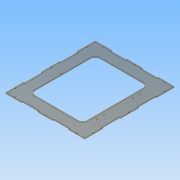
# Autodesk Inventor part: крышка
Saved by Autodesk Inventor 2017 (Build 210142000, 142)
## iProperties
Part Number: крышка
Material: Типовые
Document SubType Name: Modeling
Designer: Max
Mass: 263.553 g
Surface Area: 1424.23 cm^2
Volume: 263.553 cm^3
Density: 1 g/cm^3
Appearance: Поликарбонат — дымчатый
Author: Max
Autodesk Inventor part; units mm, degrees
ref_plane "YZ Plane" through (0, 0, 0) normal (1, 0, 0) x (0, 1, 0)
ref_plane "XZ Plane" through (0, 0, 0) normal (0, 1, 0) x (-1, 0, 0)
ref_plane "XY Plane" through (0, 0, 0) normal (0, 0, 1) x (1, 0, 0)
sketch "Эскиз1" plane through (0, 0, 0) normal (0, 0, 1) x (1, 0, 0)
  line L0 (46, -47) -> (277, -47)
  line L1 (277, -47) -> (277, -333)
  line L2 (277, -333) -> (46, -333)
  line L3 (46, -333) -> (46, -47)
  line L4 (-2, 5) -> (334, 5) projected
  line L5 (338, 5) -> (338, -385) projected
  line L6 (334, -385) -> (-2, -385) projected
  line L7 (-6, -385) -> (-6, 5) projected
  line L8 (-6, 5) -> (338, 5)
  line L9 (338, 5) -> (338, -385)
  line L10 (338, -385) -> (-6, -385)
  line L11 (-6, -385) -> (-6, 5)
  dimension "d4" = 231
  dimension "d10" = 61
  dimension "d11" = 52
  dimension "d12" = 52
  dimension "d13" = 52
  constraints: 16 end point, 4 parallel, 2 horizontal, 2 perpendicular
  measures "d4" distance between parallel lines of L1 L3
  measures "d10" distance between parallel lines of L5 L1
  measures "d11" distance between parallel lines of L4 L0
  measures "d12" distance between parallel lines of L6 L2
  measures "d13" distance between parallel lines of L7 L3
extrude "Выдавливание3" add sketch "Эскиз1" along normal blind 4
sketch "Эскиз3" plane through (0, 0, 4) normal (0, 0, 1) x (1, 0, 0)
  circle A0 centre (290.75, -97) radius 1.5
  circle A1 centre (290.75, -127) radius 1.5
  line L0 (46, -47) -> (277, -47) projected
  line L1 (277, -47) -> (277, -333) projected
  circle A2 centre (290.75, -253) radius 1.5
  circle A3 centre (290.75, -283) radius 1.5
  line L2 (277, -333) -> (46, -333) projected
  point P0 (0, 0)
  dimension "d19" = 3
  dimension "d20" = 3
  dimension "d21" = 30
  dimension "d22" = 50
  dimension "d23" = 13.75
  dimension "d24" = 13.75
  dimension "d25" = 3
  dimension "d26" = 3
  dimension "d27" = 30
  dimension "d28" = 13.75
  dimension "d29" = 13.75
  dimension "d30" = 50
  constraints: 4 centre point
  measures "d19" diameter of A0
  measures "d20" diameter of A1
  measures "d21" distance of A1.centre A0.centre
  measures "d22" distance from line of L0 A0.centre
  measures "d23" distance from line of L1 A0.centre
  measures "d24" distance from line of L1 A1.centre
  measures "d25" diameter of A2
  measures "d26" diameter of A3
  measures "d27" distance of A3.centre A2.centre
  measures "d28" distance from line of L1 A2.centre
  measures "d29" distance from line of L1 A3.centre
  measures "d30" distance from line of L2 A3.centre
extrude "Выдавливание4" cut sketch "Эскиз3" against normal blind 10
chamfer "Фаска1" distance 15 angle 45 4 edges at (277, -47, 2) (277, -333, 2) (46, -47, 2) (46, -333, 2)
sketch "Эскиз4" plane through (0, 0, 4) normal (0, 0, 1) x (1, 0, 0)
  ellipse E0 centre (40.9735, -191.8546) end of major axis (40.9735, -190.3546) minor radius 1.4997 projected
  line L0 (40.9735, -191.8546) -> (10.6659, -191.8546) construction
  circle A0 centre (40.733, -191.8546) radius 1.5
  line L1 (46, -62) -> (46, -318) projected
  point P0 (0, 0)
  dimension "d36" = 3
  dimension "d37" = 5.267
  constraints: 2 end point, 1 centre point, 1 horizontal, 1 point on line, 1 other
  measures "d36" diameter of A0
  measures "d37" distance from line of L1 A0.centre
extrude "Выдавливание5" cut sketch "Эскиз4" against normal blind 10 contours A0 E0 | E0 A0 picked at (41.2979, -191.9775) picked at (39.4227, -191.6148)
sketch "Эскиз5" plane through (0, 0, 4) normal (0, 0, 1) x (1, 0, 0)
  line L0 (-6, -73.3) -> (-2, -73.3) projected
  line L1 (-6, -150.7) -> (-2, -150.7) projected
  line L2 (-2, -73.3) -> (-2, -150.7) projected
  line L3 (-6, 5) -> (-6, -385) projected
  line L4 (-6, -229.3) -> (-2, -229.3) projected
  line L5 (-2, -229.3) -> (-2, -306.7) projected
  line L6 (-6, -306.7) -> (-2, -306.7) projected
  line L7 (63.3, -385) -> (63.3, -381) projected
  line L8 (133.2, -385) -> (63.3, -385) projected
  line L9 (133.2, -385) -> (133.2, -381) projected
  line L10 (63.3, -381) -> (133.2, -381) projected
  line L11 (63.3, -385) -> (63.3, -381) projected
  line L12 (268.7, -385) -> (198.8, -385) projected
  line L13 (268.7, -385) -> (268.7, -381) projected
  line L14 (198.8, -381) -> (268.7, -381) projected
  line L15 (198.8, -385) -> (198.8, -381) projected
  line L16 (63.3, 5) -> (133.2, 5) projected
  line L17 (63.3, 5) -> (63.3, 1) projected
  line L18 (133.2, 1) -> (63.3, 1) projected
  line L19 (133.2, 5) -> (133.2, 1) projected
  line L20 (198.8, 5) -> (268.7, 5) projected
  line L21 (198.8, 5) -> (198.8, 1) projected
  line L22 (268.7, 1) -> (198.8, 1) projected
  line L23 (268.7, 5) -> (268.7, 1) projected
  line L24 (338, -229.3) -> (334, -229.3) projected
  line L25 (334, -306.7) -> (334, -229.3) projected
  line L26 (338, -306.7) -> (334, -306.7) projected
  line L27 (338, -229.3) -> (338, -306.7) projected
  line L28 (338, -150.7) -> (334, -150.7) projected
  line L29 (338, -73.3) -> (338, -150.7) projected
  line L30 (334, -150.7) -> (334, -73.3) projected
  line L31 (338, -73.3) -> (334, -73.3) projected
  line L32 (63.1, 0.8) -> (63.1, 5.2)
  line L33 (63.1, 5.2) -> (133.4, 5.2)
  line L34 (133.4, 5.2) -> (133.4, 0.8)
  line L35 (133.4, 0.8) -> (63.1, 0.8)
  line L36 (198.6, 0.8) -> (198.6, 5.2)
  line L37 (198.6, 5.2) -> (268.9, 5.2)
  line L38 (268.9, 5.2) -> (268.9, 0.8)
  line L39 (268.9, 0.8) -> (198.6, 0.8)
  line L40 (333.8, -73.1) -> (333.8, -150.9)
  line L41 (333.8, -150.9) -> (338.2, -150.9)
  line L42 (338.2, -150.9) -> (338.2, -73.1)
  line L43 (338.2, -73.1) -> (333.8, -73.1)
  line L44 (333.8, -229.1) -> (338.2, -229.1)
  line L45 (338.2, -229.1) -> (338.2, -306.9)
  line L46 (338.2, -306.9) -> (333.8, -306.9)
  line L47 (333.8, -306.9) -> (333.8, -229.1)
  line L48 (268.9, -380.8) -> (268.9, -385.2)
  line L49 (268.9, -385.2) -> (198.6, -385.2)
  line L50 (198.6, -385.2) -> (198.6, -380.8)
  line L51 (198.6, -380.8) -> (268.9, -380.8)
  line L52 (133.2, -385) -> (63.3, -385) projected
  line L53 (133.2, -385) -> (133.2, -381) projected
  line L54 (63.3, -381) -> (133.2, -381) projected
  line L55 (63.3, -385) -> (63.3, -381) projected
  line L56 (63.3, -385) -> (63.3, -381) projected
  line L57 (63.3, -381) -> (133.2, -381) projected
  line L58 (-6, -306.9) -> (-1.8, -306.9)
  line L59 (-1.8, -306.9) -> (-1.8, -229.1)
  line L60 (-1.8, -229.1) -> (-6, -229.1)
  line L61 (-6, -150.9) -> (-1.8, -150.9)
  line L62 (-1.8, -150.9) -> (-1.8, -73.1)
  line L63 (-1.8, -73.1) -> (-6, -73.1)
  line L64 (-6, -73.1) -> (-6, -150.9)
  line L65 (-6, -229.1) -> (-6, -306.9)
  line L66 (63.3, -381) -> (133.2, -381)
  line L67 (133.2, -381) -> (133.2, -385)
  line L68 (133.2, -385) -> (63.3, -385)
  line L69 (63.3, -385) -> (63.3, -381)
  line L70 (63.3, -380.8) -> (133.2, -380.8)
  line L71 (63.1, -385) -> (63.1, -381)
  line L72 (133.4, -385) -> (133.4, -381)
  line L73 (133.4, -380.8) -> (63.1, -380.8)
  line L74 (63.1, -380.8) -> (63.1, -385.2)
  line L75 (63.1, -385.2) -> (133.4, -385.2)
  line L76 (133.4, -385.2) -> (133.4, -380.8)
  point P0 (0, 0)
  dimension "d40" = 4
  dimension "d41" = 69.9
  dimension "d42" = 69.9
  dimension "d43" = 0.2
  dimension "d44" = 0.2
  dimension "d45" = 0.2
  dimension "d46" = 0.2
  dimension "d47" = 0.2
  dimension "d48" = 0.2
  dimension "d49" = 0.2
  dimension "d50" = 0.2
  dimension "d51" = 0.2
  dimension "d52" = 0.2
  constraints: 78 end point, 7 parallel, 2 collinear, 2 horizontal, 2 perpendicular, 19 other
  measures "d40" distance between parallel lines of L18 L16
  measures "d41" distance between parallel lines of L19 L17
  measures "d42" distance between parallel lines of L23 L21
  measures "d43" distance between parallel lines of L18 L35
  measures "d44" distance between parallel lines of L21 L36
  measures "d45" distance between parallel lines of L30 L40
  measures "d46" distance between parallel lines of L25 L47
  measures "d47" distance between parallel lines of L14 L51
  measures "d48" distance between parallel lines of L6 L58
  measures "d49" distance between parallel lines of L1 L61
  measures "d50" distance between parallel lines of L10 L70
  measures "d51" distance between parallel lines of L7 L71
  measures "d52" distance between parallel lines of L9 L72
extrude "Выдавливание6" cut sketch "Эскиз5" against normal blind 4.2 contours L3 L63 L62 L61 L1 L2 L0 | L60 L59 L58 L3 L6 L5 L4 | L0 L2 L1 L3 | L4 L5 L6 L3 | L7 L10 L9 L8 | L12 L15 L14 L13 | L16 L19 L18 L17 | L20 L23 L22 L21 | L27 L26 L25 L24 | L28 L30 L31 L29 | L32 L33 L34 L35 | L36 L37 L38 L39 | L43 L42 L41 L40 | L44 L45 L46 L47 | L48 L49 L50 L51 | L70 L73 L76 L72 L75 L74 L71
sketch "Эскиз6" plane through (0, 0, 4) normal (0, 0, 1) x (1, 0, 0)
  line L0 (302.85, -381) -> (302.85, -385) projected
  line L1 (299.85, -385) -> (299.85, -381) projected
  line L2 (167.5, -381) -> (167.5, -385) projected
  line L3 (164.5, -385) -> (164.5, -381) projected
  line L4 (32.15, -381) -> (32.15, -385) projected
  line L5 (29.15, -385) -> (29.15, -381) projected
  line L6 (301.35, -381) -> (301.35, -381)
  line L7 (166, -381) -> (166, -381)
  line L8 (30.65, -381) -> (30.65, -381)
  line L9 (63.1, -380.8) -> (133.4, -380.8) projected
  line L10 (302.85, -381) -> (299.85, -381)
  line L11 (299.85, -382.5) -> (299.85, -385)
  line L12 (299.85, -385) -> (302.85, -385)
  line L13 (302.85, -385) -> (302.85, -382.5)
  line L14 (167.5, -381) -> (164.5, -381)
  line L15 (164.5, -382.5) -> (164.5, -385)
  line L16 (164.5, -385) -> (167.5, -385)
  line L17 (167.5, -385) -> (167.5, -382.5)
  line L18 (32.15, -381) -> (29.15, -381)
  line L19 (29.15, -382.5) -> (29.15, -385)
  line L20 (29.15, -385) -> (32.15, -385)
  line L21 (32.15, -385) -> (32.15, -382.5)
  line L22 (334, -344.35) -> (338, -344.35) projected
  line L23 (338, -347.35) -> (334, -347.35) projected
  line L24 (334, -188.5) -> (338, -188.5) projected
  line L25 (338, -191.5) -> (334, -191.5) projected
  line L26 (334, -32.65) -> (338, -32.65) projected
  line L27 (338, -35.65) -> (334, -35.65) projected
  line L28 (302.85, 5) -> (302.85, 1) projected
  line L29 (299.85, 1) -> (299.85, 5) projected
  line L30 (167.5, 5) -> (167.5, 1) projected
  line L31 (164.5, 1) -> (164.5, 5) projected
  line L32 (32.15, 5) -> (32.15, 1) projected
  line L33 (29.15, 1) -> (29.15, 5) projected
  line L34 (-6, -32.65) -> (-2, -32.65) projected
  line L35 (-2, -35.65) -> (-6, -35.65) projected
  line L36 (-6, -188.5) -> (-2, -188.5) projected
  line L37 (-2, -191.5) -> (-6, -191.5) projected
  line L38 (-6, -344.35) -> (-2, -344.35) projected
  line L39 (-2, -347.35) -> (-6, -347.35) projected
  line L40 (338, -344.35) -> (335.5, -344.35)
  line L41 (334, -345.85) -> (334, -345.85)
  line L42 (335.5, -347.35) -> (338, -347.35)
  line L43 (338, -347.35) -> (338, -344.35)
  line L44 (338, -188.5) -> (335.5, -188.5)
  line L45 (334, -190) -> (334, -190)
  line L46 (335.5, -191.5) -> (338, -191.5)
  line L47 (338, -191.5) -> (338, -188.5)
  line L48 (338, -32.65) -> (335.5, -32.65)
  line L49 (334, -34.15) -> (334, -34.15)
  line L50 (335.5, -35.65) -> (338, -35.65)
  line L51 (338, -35.65) -> (338, -32.65)
  line L52 (302.85, 5) -> (299.85, 5)
  line L53 (299.85, 5) -> (299.85, 2.5)
  line L54 (301.35, 1) -> (301.35, 1)
  line L55 (302.85, 2.5) -> (302.85, 5)
  line L56 (167.5, 5) -> (164.5, 5)
  line L57 (164.5, 5) -> (164.5, 2.5)
  line L58 (166, 1) -> (166, 1)
  line L59 (167.5, 2.5) -> (167.5, 5)
  line L60 (32.15, 5) -> (29.15, 5)
  line L61 (29.15, 5) -> (29.15, 2.5)
  line L62 (30.65, 1) -> (30.65, 1)
  line L63 (32.15, 2.5) -> (32.15, 5)
  line L64 (-3.5, -32.65) -> (-6, -32.65)
  line L65 (-6, -32.65) -> (-6, -35.65)
  line L66 (-6, -35.65) -> (-3.5, -35.65)
  line L67 (-2, -34.15) -> (-2, -34.15)
  line L68 (-3.5, -188.5) -> (-6, -188.5)
  line L69 (-6, -188.5) -> (-6, -191.5)
  line L70 (-6, -191.5) -> (-3.5, -191.5)
  line L71 (-2, -190) -> (-2, -190)
  line L72 (-3.5, -344.35) -> (-6, -344.35)
  line L73 (-6, -344.35) -> (-6, -347.35)
  line L74 (-6, -347.35) -> (-3.5, -347.35)
  line L75 (-2, -345.85) -> (-2, -345.85)
  arc A0 (167.5, -382.5) -> (166, -381) centre (166, -382.5) ccw
  arc A1 (166, -381) -> (164.5, -382.5) centre (166, -382.5) ccw
  arc A2 (32.15, -382.5) -> (30.65, -381) centre (30.65, -382.5) ccw
  arc A3 (30.65, -381) -> (29.15, -382.5) centre (30.65, -382.5) ccw
  arc A4 (-2, -345.85) -> (-3.5, -344.35) centre (-3.5, -345.85) ccw
  arc A5 (-3.5, -347.35) -> (-2, -345.85) centre (-3.5, -345.85) ccw
  arc A6 (-2, -190) -> (-3.5, -188.5) centre (-3.5, -190) ccw
  arc A7 (-3.5, -191.5) -> (-2, -190) centre (-3.5, -190) ccw
  arc A8 (-2, -34.15) -> (-3.5, -32.65) centre (-3.5, -34.15) ccw
  arc A9 (-3.5, -35.65) -> (-2, -34.15) centre (-3.5, -34.15) ccw
  arc A10 (30.65, 1) -> (32.15, 2.5) centre (30.65, 2.5) ccw
  arc A11 (29.15, 2.5) -> (30.65, 1) centre (30.65, 2.5) ccw
  arc A12 (166, 1) -> (167.5, 2.5) centre (166, 2.5) ccw
  arc A13 (164.5, 2.5) -> (166, 1) centre (166, 2.5) ccw
  arc A14 (301.35, 1) -> (302.85, 2.5) centre (301.35, 2.5) ccw
  arc A15 (299.85, 2.5) -> (301.35, 1) centre (301.35, 2.5) ccw
  arc A16 (335.5, -32.65) -> (334, -34.15) centre (335.5, -34.15) ccw
  arc A17 (334, -34.15) -> (335.5, -35.65) centre (335.5, -34.15) ccw
  arc A18 (335.5, -188.5) -> (334, -190) centre (335.5, -190) ccw
  arc A19 (334, -190) -> (335.5, -191.5) centre (335.5, -190) ccw
  arc A20 (335.5, -344.35) -> (334, -345.85) centre (335.5, -345.85) ccw
  arc A21 (334, -345.85) -> (335.5, -347.35) centre (335.5, -345.85) ccw
  arc A22 (302.85, -382.5) -> (301.35, -381) centre (301.35, -382.5) ccw
  arc A23 (301.35, -381) -> (299.85, -382.5) centre (301.35, -382.5) ccw
  point P0 (0, 0)
  dimension "d55" = 1.5
  dimension "d56" = 1.5
  constraints: 102 end point, 48 point on circle, 48 tangent, 30 point on line, 25 parallel, 24 centre point, 22 equal radius, 14 perpendicular, 12 horizontal
  measures "d55" radius of A0
  measures "d56" radius of A2
extrude "Выдавливание7" cut sketch "Эскиз6" against normal blind 10 contours L0 L12 L1 A23 A22 | L2 L16 L3 A1 A0 | L4 L20 L5 A3 A2 | L22 L43 L23 A21 A20 | L24 L47 L25 A19 A18 | L26 L51 L27 A17 A16 | L28 A14 A15 L29 L52 | L30 A12 A13 L31 L56 | L32 A10 A11 L33 L60 | L34 A8 A9 L35 L65 | L36 A6 A7 L37 L69 | L38 A4 A5 L39 L73
